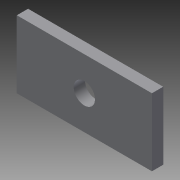
# Autodesk Inventor part: CURM_Caterpillar_Tail
Saved by Autodesk Inventor 2015 (Build 190159000, 159)
## iProperties
Created: 2015-02-13
Part Number: CURM_Caterpillar_Tail
Material: Generic
Document SubType Name: Modeling
Designer: Judson
Density: 1 g/cm^3
Appearance: Default
Author: Judson
Autodesk Inventor part; units mm, degrees
ref_plane "YZ Plane" through (0, 0, 0) normal (1, 0, 0) x (0, 1, 0)
ref_plane "XZ Plane" through (0, 0, 0) normal (0, 1, 0) x (-1, 0, 0)
ref_plane "XY Plane" through (0, 0, 0) normal (0, 0, 1) x (1, 0, 0)
sketch "Sketch1" plane through (0, 0, 0) normal (0, 0, 1) x (1, 0, 0)
  line L0 (-15.6535, 8.2698) -> (22.4465, 8.2698)
  line L1 (22.4465, 8.2698) -> (22.4465, -10.7802)
  line L2 (22.4465, -10.7802) -> (-15.6535, -10.7802)
  line L3 (-15.6535, -10.7802) -> (-15.6535, 8.2698)
  circle A0 centre (3.3965, -1.2552) radius 3
  point P0 (0, 0)
  dimension "d0" = 38.1
  dimension "d1" = 19.05
  dimension "d4" = 6
  constraints: 8 end point, 2 parallel, 1 centre point, 1 horizontal, 1 perpendicular
  measures "d0" distance of L1.end L2.end
  measures "d1" distance of L2.end L0.start
  measures "d4" diameter of A0
extrude "Extrusion1" add sketch "Sketch1" along normal blind 3.175 contours L0 L1 L2 L3 | A0
extrude "Extrusion2" cut sketch "Sketch1" along normal blind 3.175 contours A0
body "Solid1"
